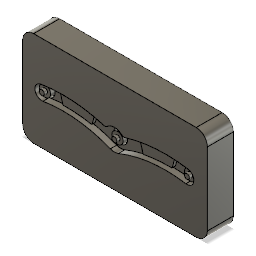
3.5 Draft (Autodesk Fusion 360 design; units mm, degrees)
Autodesk Fusion 360 part; units mm, degrees
note: some values were not read from the file. Set by a fixed rule: which sketch regions a step uses.
sketch "Sketch1" plane through (0, 0, 0) normal (0, 0, 1) x (1, 0, 0)
  circle A0 centre (0, 0) radius 4
  circle A1 centre (0, 0) radius 9
  circle A2 centre (0, 0) radius 11
  circle A3 centre (115, 7) radius 4
  circle A4 centre (115, 7) radius 9
  arc A5 (113.2342, -3.8573) -> (6.3557, -15.7672) centre (81.1291, -201.2637) ccw
  circle A6 centre (115, 7) radius 11
  arc A7 (85.785, 1.6829) -> (41.4288, -2.1836) centre (81.1291, -201.2637) ccw
  arc A8 (89.5687, 17.5736) -> (37.4029, 13.3267) centre (81.1291, -201.2637) ccw
  arc A9 (116.7658, 17.8573) -> (16.6159, 11.1558) centre (81.1291, -201.2637) ccw
  line L0 (115, 7) -> (88, 7) construction
  line L1 (88, 7) -> (38, 7) construction
  line L2 (90.4961, 16.3156) -> (86.7738, 2.4238)
  line L3 (36.6367, 12.088) -> (40.2673, -1.4617)
  arc A10 (37.4029, 13.3267) -> (36.6367, 12.088) centre (37.6026, 12.3468) ccw
  arc A11 (40.2673, -1.4617) -> (41.4288, -2.1836) centre (41.2332, -1.2029) ccw
  arc A12 (90.4961, 16.3156) -> (89.5687, 17.5736) centre (89.5302, 16.5744) ccw
  arc A13 (85.785, 1.6829) -> (86.7738, 2.4238) centre (85.8079, 2.6827) ccw
  line L4 (0, 0) -> (0, -43.0721) construction
  circle A14 centre (-115, 7) radius 4
  arc A15 (-6.3557, -15.7672) -> (-113.2342, -3.8573) centre (-81.1291, -201.2637) ccw
  arc A16 (-16.6159, 11.1558) -> (-116.7658, 17.8573) centre (-81.1291, -201.2637) ccw
  arc A17 (-41.4288, -2.1836) -> (-85.785, 1.6829) centre (-81.1291, -201.2637) ccw
  arc A18 (-37.4029, 13.3267) -> (-89.5687, 17.5736) centre (-81.1291, -201.2637) ccw
  arc A19 (-89.5687, 17.5736) -> (-90.4961, 16.3156) centre (-89.5302, 16.5744) ccw
  circle A20 centre (-115, 7) radius 9
  arc A21 (-86.7738, 2.4238) -> (-85.785, 1.6829) centre (-85.8079, 2.6827) ccw
  line L5 (-115, 7) -> (-88, 7) construction
  line L6 (-36.6367, 12.088) -> (-40.2673, -1.4617)
  arc A22 (-41.4288, -2.1836) -> (-40.2673, -1.4617) centre (-41.2332, -1.2029) ccw
  circle A23 centre (-115, 7) radius 11
  line L7 (-90.4961, 16.3156) -> (-86.7738, 2.4238)
  arc A24 (-36.6367, 12.088) -> (-37.4029, 13.3267) centre (-37.6026, 12.3468) ccw
  line L8 (-88, 7) -> (-38, 7) construction
  arc A25 (-6.3557, -15.7672) -> (6.3557, -15.7672) centre (0, 0) ccw
  arc A26 (11.7168, 12.3173) -> (-11.7168, 12.3173) centre (0, 0) ccw
  arc A27 (-16.6159, 11.1558) -> (-11.7168, 12.3173) centre (-15.1629, 15.9401) ccw
  arc A28 (11.7168, 12.3173) -> (16.6159, 11.1558) centre (15.1629, 15.9401) ccw
  dimension "d1" = 18
  dimension "d2" = 22
  dimension "d3" = 18
  dimension "d5" = 34
  dimension "d14" = 8
  dimension "d15" = 22
  dimension "d16" = 8
  dimension "d17" = 7
  dimension "d18" = 115
  dimension "d19" = 200
  dimension "d23" = 27
  dimension "d24" = 50
  dimension "d25" = 75
  dimension "d26" = 75
  dimension "d27" = 1
  dimension "d28" = 1
  dimension "d29" = 1
  dimension "d30" = 1
  dimension "d31" = 3
  dimension "d32" = 3
  dimension "d33" = 5
  dimension "d34" = 5
  measures "d1" diameter of A1
  measures "d2" diameter of A2
  measures "d3" diameter of A4
  measures "d5" diameter of A25
  measures "d14" diameter of A0
  measures "d15" diameter of A6
  measures "d16" diameter of A3
  measures "d17" distance of A0.centre
  measures "d18" distance of A0.centre
  measures "d19" radius of A5
  measures "d25" angle of L0 L2
  measures "d26" angle of L1 L3
  measures "d27" radius of A10
  measures "d28" radius of A11
  measures "d29" radius of A12
  measures "d30" radius of A13
  measures "d31" distance of A5 A7
  measures "d32" distance of A8 A9
  measures "d33" radius of A27
  measures "d34" radius of A28
extrude "Extrude1" add sketch "Sketch1" along normal mid plane 20 contours A5 A6 A9 A15 A16 A23 A25 A26 A27 A28 makes body 1
extrude "Extrude2" add sketch "Sketch1" along normal mid plane 10 contours A7 A8 L2 L3 A10 A11 A12 A13 | A17 A18 A19 A21 L6 A22 L7 A24 bodies 1
extrude "Extrude3" add sketch "Sketch1" along normal mid plane 32 contours A2 | A6 | A23 bodies 1
extrude "Extrude4" add sketch "Sketch1" along normal mid plane 10 contours A1 | A4 | A20 bodies 1
sketch "Sketch2" plane through (0, 0, 0) normal (0, 0, 1) x (1, 0, 0)
  line L0 (-127.8859, 81.5623) -> (129.7008, 81.5623)
  line L1 (147.4554, 63.8076) -> (147.4554, -51.5592)
  line L2 (129.7008, -69.3138) -> (-127.8859, -69.3138)
  line L3 (-145.6405, -51.5592) -> (-145.6405, 63.8076)
  arc A0 (-127.8859, 81.5623) -> (-145.6405, 63.8076) centre (-127.8859, 63.8076) ccw
  arc A1 (-145.6405, -51.5592) -> (-127.8859, -69.3138) centre (-127.8859, -51.5592) ccw
  arc A2 (129.7008, -69.3138) -> (147.4554, -51.5592) centre (129.7008, -51.5592) ccw
  arc A3 (147.4554, 63.8076) -> (129.7008, 81.5623) centre (129.7008, 63.8076) ccw
  dimension "d47" = 17.7546
  measures "d47" radius of A0
extrude "Extrude5" add sketch "Sketch2" against normal blind 41.381 separate body makes body 2
combine "Combine1" operation cut target body 2 tool bodies 1
